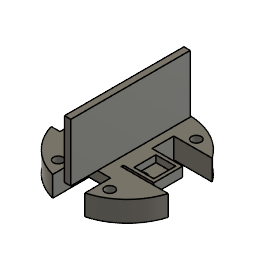
TwoSiPM_Metalens_Holder (Autodesk Fusion 360 design; units mm, degrees)
part number: 2026-07-10-10-46-46-883
Autodesk Fusion 360 part; units mm, degrees
note: some values were not read from the file. Set by a fixed rule: which sketch regions a step uses.
sketch "Sketch Base" plane through (0, 0, 0) normal (0, 1, 0) x (1, 0, 0)
  circle A0 centre (0, 0) radius 19
  line L0 (-4.9826, -7.0157) -> (5.0174, -6.9909)
  line L1 (-4.9826, -7.0157) -> (-4.9545, -18.3427)
  line L2 (5.0174, -6.9909) -> (5.0455, -18.3178)
  line L3 (3.5525, 10.9149) -> (15.552, 10.9149)
  line L4 (-3.5525, 10.9149) -> (-15.552, 10.9149)
  line L5 (3.5525, -5.4945) -> (18.1991, -5.4582)
  line L6 (-3.5525, -5.5769) -> (-18.1631, -5.5769)
  line L7 (3.5525, -5.4945) -> (3.5525, 10.9149)
  line L8 (-3.5525, -5.5769) -> (-3.5525, 10.9149)
  dimension "d1" = 38
  dimension "d4" = 10
  dimension "d10" = 1.5
  dimension "d11" = 7.105
  dimension "d31" = 11.327
  constraint coincident A0.centre origin
  constraint coincident A0 L1.end
  constraint perpendicular L0 L1
  constraint coincident A0 L2.end
  constraint perpendicular L0 L2
  constraint coincident A0 L3.end
  constraint coincident A0 L4.end
  constraint coincident A0 L5.end
  constraint coincident A0 L6.end
  constraint perpendicular L3 L7
  constraint perpendicular L4 L8
  constraint equal L1 L2
  measures "d1" diameter of A0
  measures "d4" distance of L0.start L0.end
  measures "d10" distance of L0 L5
  measures "d11" distance of L7 L8
  measures "d31" distance of L0.start L1.end
extrude "Extrude Base" add sketch "Sketch Base" along normal blind 6.45 contours A0 L0 L1 L2 L3 L4 L5 L6 L7 L8
sketch "Sketch Middle Separations" plane through (0, 6.45, 0) normal (0, 1, 0) x (-1, 0, 0)
  arc A0 (18.1631, 5.5769) -> (4.9545, 18.3427) centre (0, 0) ccw
  line L0 (4.9545, 18.3427) -> (4.9826, 7.0157)
  line L1 (4.9826, 7.0157) -> (-5.0174, 6.9909)
  line L2 (-5.0174, 6.9909) -> (-5.0455, 18.3178)
  arc A1 (-5.0455, 18.3178) -> (-18.1991, 5.4582) centre (0, 0) ccw
  line L3 (-18.1991, 5.4582) -> (-3.5525, 5.4945)
  line L4 (-3.5525, 5.4945) -> (-3.5525, -10.9149)
  line L5 (-3.5525, -10.9149) -> (-15.552, -10.9149)
  arc A2 (-15.552, -10.9149) -> (15.552, -10.9149) centre (0, 0) ccw
  line L6 (15.552, -10.9149) -> (3.5525, -10.9149)
  line L7 (3.5525, -10.9149) -> (3.5525, 5.5769)
  line L8 (3.5525, 5.5769) -> (18.1631, 5.5769)
  line L9 (1, 18.6355) -> (-1, 18.6355)
  line L10 (-1, 18.6355) -> (-1, -18.6355)
  line L11 (1, 18.6355) -> (1, -18.6355)
  line L12 (-1, -18.6355) -> (1, -18.6355)
  line L13 (1, -18.6355) -> (2.1, -18.6355)
  line L14 (2.1, -18.6355) -> (2.1, 10.3085)
  line L15 (2.1, 10.3085) -> (1, 10.3085)
  line L16 (-2.1, -18.6355) -> (-1, -18.6355)
  line L17 (-2.1, -18.6355) -> (-2.1, 10.3085)
  line L18 (-2.1, 10.3085) -> (-1, 10.3085)
  dimension "d15" = 2
  dimension "d16" = 37.271
  dimension "d32" = 28.944
  dimension "d100" = 1.1
  dimension "d114" = 1.1
  constraint perpendicular L9 L10
  constraint perpendicular L9 L11
  constraint equal L10 L11
  constraint perpendicular L11 L13
  constraint perpendicular L13 L14
  constraint coincident L11 L15.end
  constraint perpendicular L11 L15
  constraint perpendicular L10 L16
  constraint perpendicular L5 L17
  constraint coincident L10 L18.end
  constraint perpendicular L10 L18
  constraint equal L14 L17
  measures "d15" distance of L9.start L9.end
  measures "d16" distance of L9.end L10.end
  measures "d32" distance of L16.start L17.end
  measures "d100" distance of L17.end L18.end
  measures "d114" distance of L14.end L15.end
extrude "Extrude Middle Separations" add sketch "Sketch Middle Separations" along normal blind 18 contours L1 L10 L11 L12 | L1 L9 L10 L11
sketch "Sketch Aesthetic" plane through (0.0174, 0, 7.0033) normal (0.002481, 0, 0.999997) x (0.999997, 0, -0.002481)
  line L0 (-5, 0) -> (5, 0)
  line L1 (5, 0) -> (5, 6.45)
  line L2 (5, 6.45) -> (0.9826, 6.45)
  line L3 (0.9826, 6.45) -> (-1.0174, 6.45)
  line L4 (-1.0174, 6.45) -> (-5, 6.45)
  line L5 (-5, 6.45) -> (-5, 0)
  line L6 (5, 6.45) -> (5, 3.35)
  line L7 (5, 3.35) -> (-5, 3.35)
  line L8 (-5, 3.35) -> (-5, 6.45)
  line L9 (5, 6.45) -> (-5, 6.45)
  dimension "d28" = 3.1
  constraint coincident L1.end L2.start
  constraint perpendicular L2 L6
  constraint coincident L5 L7.end
  constraint perpendicular L5 L7
  constraint coincident L4.end L5.start
  measures "d28" distance of L1.end L6.end
extrude "Extrude Aesthetic" add sketch "Sketch Aesthetic" along normal blind 3.3 contours L1 L2 L3 L4 L5 L6 L7 L8 L9
sketch "Sketch 6x6 SiPM Holder" plane through (-3.5525, 0, 0) normal (-1, 0, 0) x (0, 0, 1)
  line L0 (5.5769, 3.45) -> (-5.5301, 3.45)
  line L1 (-5.5301, 3.45) -> (-5.5301, 6.45)
  line L2 (-5.5301, 6.45) -> (5.5769, 6.45)
  line L3 (5.5769, 6.45) -> (5.5769, 3.45)
  line L4 (-10.9149, 0) -> (5.5769, 0)
  line L5 (5.5769, 0) -> (5.5769, 6.45)
  line L6 (5.5769, 6.45) -> (-10.9149, 6.45)
  line L7 (-10.9149, 6.45) -> (-10.9149, 0)
  dimension "d135" = 3
  dimension "d136" = 11.107
  constraint horizontal L0
  constraint vertical L1
  constraint horizontal L2
  constraint vertical L3
  constraint coincident L2.end L6
  constraint coincident L2.end L3.start
  measures "d135" distance of L0.start L2.end
  measures "d136" distance of L0.start L0.end
extrude "Extrude 6x6 SiPM Holder" add sketch "Sketch 6x6 SiPM Holder" along normal blind 11.884 contours L0 L1 L2 L3 L5 L6
sketch "Sketch 6x6 SiPM Holder Bis" plane through (0, 6.45, 0) normal (0, 1, 0) x (-1, 0, 0)
  line L0 (3.5525, -5.5301) -> (15.4365, -5.5301)
  line L1 (15.4365, -5.5301) -> (15.4365, 5.5769)
  line L2 (14.3365, -4.4301) -> (3.5525, -4.4301)
  line L3 (3.5525, -4.4301) -> (3.5525, 4.6399)
  line L4 (3.5525, 4.6399) -> (14.3365, 4.6399)
  line L5 (14.3365, 4.6399) -> (14.3365, -4.4301)
  line L6 (1, -18.6355) -> (-1, -18.6355)
  line L7 (-1, 10.3009) -> (-5.0256, 10.2909)
  line L8 (-5.0256, 10.2909) -> (-5.0455, 18.3178)
  arc A0 (-5.0455, 18.3178) -> (-18.1991, 5.4582) centre (0, 0) ccw
  line L9 (-18.1991, 5.4582) -> (-3.5525, 5.4945)
  line L10 (-3.5525, 5.4945) -> (-3.5525, -10.9149)
  line L11 (-3.5525, -10.9149) -> (-15.552, -10.9149)
  arc A1 (-15.552, -10.9149) -> (15.552, -10.9149) centre (0, 0) ccw
  line L12 (15.552, -10.9149) -> (3.5525, -10.9149)
  line L13 (3.5525, -10.9149) -> (3.5525, -5.5301)
  line L14 (15.4365, 5.5769) -> (18.1631, 5.5769)
  arc A2 (18.1631, 5.5769) -> (4.9545, 18.3427) centre (0, 0) ccw
  line L15 (4.9545, 18.3427) -> (4.9744, 10.3157)
  line L16 (-1, -18.6355) -> (-1, 10.3009)
  line L17 (4.9744, 10.3157) -> (1, 10.3058)
  line L18 (1, 10.3058) -> (1, -18.6355)
  dimension "d142" = 9.07
  dimension "d143" = 10.784
  dimension "d144" = 1.1
  constraint horizontal L2
  constraint vertical L3
  constraint horizontal L4
  constraint vertical L5
  measures "d142" distance of L2.start L4.end
  measures "d143" distance of L3.end L4.end
  measures "d144" distance of L0 L2
extrude "Extrude 6x6 SiPM Holder Bis" cut sketch "Sketch 6x6 SiPM Holder Bis" against normal blind 2.1 contours L2 L3 L4 L5
sketch "Sketch 6x6 SiPM Legs Holes" plane through (0, 4.35, 0) normal (0, 1, 0) x (-1, 0, 0)
  line L0 (3.5525, -4.4304) -> (14.3365, -4.4304)
  line L1 (14.3365, -4.4304) -> (14.3365, 4.6396)
  line L2 (14.3365, 4.6396) -> (3.5525, 4.6396)
  line L3 (3.5525, 4.6396) -> (3.5525, -4.4304)
  circle A0 centre (5.3481, 0.1396) radius 1
  circle A1 centre (12.7861, 0.1396) radius 1
  line L4 (14.3365, 4.6399) -> (3.5525, 4.6399)
  line L5 (3.5525, 4.6399) -> (3.5525, -4.4301)
  line L6 (3.5525, -4.4301) -> (14.3365, -4.4301)
  line L7 (14.3365, -4.4301) -> (14.3365, 4.6399)
  circle A2 centre (5.3481, 2.3396) radius 1
  line L8 (4.3481, 2.3396) -> (4.3481, 0.1396)
  line L9 (6.3481, 2.3349) -> (6.3481, 0.1396)
  circle A3 centre (12.7861, 2.3396) radius 1
  line L10 (11.7861, 2.3396) -> (11.7861, 0.1396)
  line L11 (13.7861, 2.3396) -> (13.7855, 0.1046)
  dimension "d63" = 2
  dimension "d67" = 4.5
  dimension "d95" = 2
  dimension "d96" = 7.438
  dimension "d152" = 2
  dimension "d153" = 2.2
  dimension "d154" = 2.3
  dimension "d155" = 2
  constraint coincident A1 L11.end
  constraint coincident A2 L8.start
  constraint coincident A0 L8.end
  constraint tangent A0 L8
  constraint coincident A2 L9.start
  constraint coincident A0 L9.end
  constraint tangent A0 L9
  constraint coincident A3 L10.start
  constraint coincident A1 L10.end
  constraint tangent A1 L10
  constraint vertical L10
  constraint coincident A3 L11.start
  measures "d63" diameter of A0
  measures "d67" distance of L2 A0.centre
  measures "d95" diameter of A1
  measures "d96" distance of A0.centre A1.centre
  measures "d152" diameter of A2
  measures "d153" distance of A0.centre A2.centre
  measures "d154" distance of L2 A2.centre
  measures "d155" diameter of A3
extrude "Extrude 6x6 SiPM Legs Holes" cut sketch "Sketch 6x6 SiPM Legs Holes" against normal blind 1.1 contours A0 | A0 A2 L8 L9 | A2 | A1 L11 | A1 A3 L10 L11 | A3
sketch "Sketch 3x3 SiPM Holder" plane through (3.5525, 0, 0) normal (1, 0, 0) x (0, 0, -1)
  line L0 (-5.4945, 0) -> (10.9149, 0)
  line L1 (10.9149, 0) -> (10.9149, 6.45)
  line L2 (10.9149, 6.45) -> (-5.4945, 6.45)
  line L3 (-5.4945, 6.45) -> (-5.4945, 0)
  line L4 (-4.83, 6.45) -> (4.17, 6.45)
  line L5 (4.17, 6.45) -> (4.17, 3.45)
  line L6 (4.17, 3.45) -> (-4.83, 3.45)
  line L7 (-4.83, 3.45) -> (-4.83, 6.45)
  dimension "d148" = 3
  dimension "d149" = 9
  constraint horizontal L4
  constraint vertical L5
  constraint horizontal L6
  constraint vertical L7
  measures "d148" distance of L4.start L6.end
  measures "d149" distance of L5.end L6.end
extrude "Extrude 3x3 SiPM Holder (1)" add sketch "Sketch 3x3 SiPM Holder" along normal blind 9.517 contours L2 L4 L5 L6 L7
sketch "Sketch 3x3 SiPM Holder Bis" plane through (0, 6.45, 0) normal (0, 1, 0) x (-1, 0, 0)
  line L0 (2.1, 10.3085) -> (2.1, -18.6355)
  line L1 (2.1, -18.6355) -> (-2.1, -18.6355)
  line L2 (-2.1, -18.6355) -> (-2.1, 10.2981)
  line L3 (-2.1, 10.2981) -> (-5.0256, 10.2909)
  line L4 (-5.0256, 10.2909) -> (-5.0455, 18.3178)
  arc A0 (-5.0455, 18.3178) -> (-18.1991, 5.4582) centre (0, 0) ccw
  line L5 (-18.1991, 5.4582) -> (-3.5525, 5.4945)
  line L6 (-3.5525, 5.4945) -> (-3.5525, -10.9149)
  line L7 (-3.5525, -10.9149) -> (-15.552, -10.9149)
  arc A1 (-15.552, -10.9149) -> (15.552, -10.9149) centre (0, 0) ccw
  line L8 (15.552, -10.9149) -> (3.5525, -10.9149)
  line L9 (3.5525, -10.9149) -> (3.5525, 5.5769)
  line L10 (3.5525, 5.5769) -> (18.1631, 5.5769)
  arc A2 (18.1631, 5.5769) -> (4.9545, 18.3427) centre (0, 0) ccw
  line L11 (4.9545, 18.3427) -> (4.9744, 10.3157)
  line L12 (4.9744, 10.3157) -> (2.0818, 10.3085)
  line L13 (2.0818, 10.3085) -> (2.1, 10.3085)
  line L14 (-11.9695, 3.73) -> (-5.8195, 3.73)
  line L15 (-11.9695, 3.73) -> (-11.9695, -3.07)
  line L16 (-11.9695, -3.07) -> (-5.8195, -3.07)
  line L17 (-5.8195, -3.07) -> (-5.8195, 3.73)
  line L18 (-3.5525, 4.83) -> (-13.0695, 4.83)
  line L19 (-13.0695, 4.83) -> (-13.0695, -4.17)
  line L20 (-13.0695, -4.17) -> (-3.5525, -4.17)
  line L21 (-3.5525, 5.4945) -> (-3.5525, 4.83)
  line L22 (1, -18.6355) -> (-1, -18.6355)
  line L23 (-1, 10.3009) -> (-5.0256, 10.2909)
  line L24 (-5.0256, 10.2909) -> (-5.0455, 18.3178)
  arc A3 (-5.0455, 18.3178) -> (-18.1991, 5.4582) centre (0, 0) ccw
  line L25 (-18.1991, 5.4582) -> (-3.5525, 5.4945)
  line L26 (-3.5525, -4.17) -> (-3.5525, -10.9149)
  line L27 (-3.5525, -10.9149) -> (-15.552, -10.9149)
  arc A4 (-15.552, -10.9149) -> (15.552, -10.9149) centre (0, 0) ccw
  line L28 (15.552, -10.9149) -> (3.5525, -10.9149)
  line L29 (3.5525, -10.9149) -> (3.5525, -5.5301)
  line L30 (3.5525, -4.4301) -> (3.5525, 4.6399)
  line L31 (15.4365, 5.5769) -> (18.1631, 5.5769)
  arc A5 (18.1631, 5.5769) -> (4.9545, 18.3427) centre (0, 0) ccw
  line L32 (4.9545, 18.3427) -> (4.9744, 10.3157)
  line L33 (3.5525, 4.6399) -> (14.3365, 4.6399)
  line L34 (14.3365, 4.6399) -> (14.3365, -4.4301)
  line L35 (14.3365, -4.4301) -> (3.5525, -4.4301)
  line L36 (3.5525, -5.5301) -> (15.4365, -5.5301)
  line L37 (15.4365, -5.5301) -> (15.4365, 5.5769)
  line L38 (-1, -18.6355) -> (-1, 10.3009)
  line L39 (4.9744, 10.3157) -> (1, 10.3058)
  line L40 (1, 10.3058) -> (1, -18.6355)
  dimension "d78" = 6.15
  dimension "d82" = 6.8
  constraint perpendicular L15 L16
  constraint equal L14 L16
  measures "d78" distance of L14.start L14.end
  measures "d82" distance of L14.start L15.end
extrude "Extrude 3x3 SiPM Holder Bis" cut sketch "Sketch 3x3 SiPM Holder Bis" against normal blind 2.1 contours L14 L15 L16 L17
sketch "Sketch 3x3 SiPM Legs Holes" plane through (0, 4.35, 0) normal (0, 1, 0) x (-1, 0, 0)
  line L0 (-11.9695, 3.73) -> (-11.9695, -3.07)
  line L1 (-11.9695, -3.07) -> (-5.8195, -3.07)
  line L2 (-5.8195, -3.07) -> (-5.8195, 3.73)
  line L3 (-5.8195, 3.73) -> (-11.9695, 3.73)
  circle A0 centre (-10.1695, 2.33) radius 1
  circle A1 centre (-7.6195, 2.33) radius 1
  line L4 (-11.9695, 3.73) -> (-11.9695, -3.07)
  line L5 (-11.9695, -3.07) -> (-5.8195, -3.07)
  line L6 (-5.8195, -3.07) -> (-5.8195, 3.73)
  line L7 (-5.8195, 3.73) -> (-11.9695, 3.73)
  circle A2 centre (-6.8295, 2.33) radius 1
  line L8 (-7.6213, 3.33) -> (-6.8295, 3.33)
  line L9 (-7.6213, 1.33) -> (-6.8295, 1.33)
  circle A3 centre (-10.9595, 2.33) radius 1
  line L10 (-10.1684, 3.33) -> (-10.9595, 3.33)
  line L11 (-10.9595, 1.33) -> (-10.1695, 1.33)
  dimension "d85" = 2
  dimension "d87" = 2.55
  dimension "d158" = 2
  dimension "d160" = 2
  dimension "d161" = 0.79
  dimension "d162" = 0.79
  constraint coincident A1 L8.start
  constraint coincident A2 L8.end
  constraint tangent A2 L8
  constraint coincident A1 L9.start
  constraint coincident A2 L9.end
  constraint tangent A2 L9
  constraint coincident A0 L10.start
  constraint coincident A3 L10.end
  constraint tangent A3 L10
  constraint coincident A3 L11.start
  constraint coincident A0 L11.end
  constraint tangent A0 L11
  constraint horizontal L11
  measures "d85" diameter of A0
  measures "d87" horizontal distance of A0.centre A1.centre
  measures "d158" diameter of A2
  measures "d160" diameter of A3
  measures "d161" distance of A0.centre A3.centre
  measures "d162" distance of A1.centre A2.centre
extrude "Extrude 3x3 SiPM Legs Holes" cut sketch "Sketch 3x3 SiPM Legs Holes" against normal blind 1.1 contours A0 A3 L10 | A0 A3 | A0 A3 L11 | A0 A3 | A0 A3 | A1 A2 L9 | A1 A2 | A1 A2 L8 | A1 A2 | A1 A2
sketch "Sketch Base Crews Holes" plane through (0, 6.45, 0) normal (0, 1, 0) x (-1, 0, 0)
  line L0 (1, -18.6355) -> (-1, -18.6355)
  line L1 (-1, 10.3009) -> (-5.0256, 10.2909)
  line L2 (-5.0256, 10.2909) -> (-5.0455, 18.3178)
  arc A0 (-5.0455, 18.3178) -> (-18.1991, 5.4582) centre (0, 0) ccw
  line L3 (-18.1991, 5.4582) -> (-3.5525, 5.4945)
  line L4 (-3.5525, 5.4945) -> (-3.5525, 4.83)
  line L5 (-3.5525, -10.9149) -> (-15.552, -10.9149)
  arc A1 (-15.552, -10.9149) -> (15.552, -10.9149) centre (0, 0) ccw
  line L6 (15.552, -10.9149) -> (3.5525, -10.9149)
  line L7 (3.5525, -10.9149) -> (3.5525, -5.5301)
  line L8 (15.4365, 5.5769) -> (18.1631, 5.5769)
  arc A2 (18.1631, 5.5769) -> (4.9545, 18.3427) centre (0, 0) ccw
  line L9 (4.9545, 18.3427) -> (4.9744, 10.3157)
  circle A3 centre (8.0047, 13.5403) radius 1.5
  circle A4 centre (-7.9953, 13.5006) radius 1.5
  circle A5 centre (-7.9281, -13.5711) radius 1.5
  circle A6 centre (8.0719, -13.5711) radius 1.5
  line L10 (-5.8195, -3.07) -> (-11.9695, -3.07)
  line L11 (-11.9695, -3.07) -> (-11.9695, 3.73)
  line L12 (-11.9695, 3.73) -> (-5.8195, 3.73)
  line L13 (-5.8195, 3.73) -> (-5.8195, -3.07)
  line L14 (-3.5525, 4.83) -> (-13.0695, 4.83)
  line L15 (-13.0695, 4.83) -> (-13.0695, -4.17)
  line L16 (-13.0695, -4.17) -> (-3.5525, -4.17)
  line L17 (-3.5525, -4.17) -> (-3.5525, -10.9149)
  line L18 (3.5525, -4.4301) -> (3.5525, 4.6399)
  line L19 (3.5525, 4.6399) -> (14.3365, 4.6399)
  line L20 (14.3365, 4.6399) -> (14.3365, -4.4301)
  line L21 (14.3365, -4.4301) -> (3.5525, -4.4301)
  line L22 (3.5525, -5.5301) -> (15.4365, -5.5301)
  line L23 (15.4365, -5.5301) -> (15.4365, 5.5769)
  line L24 (-1, -18.6355) -> (-1, 10.3009)
  line L25 (4.9744, 10.3157) -> (1, 10.3058)
  line L26 (1, 10.3058) -> (1, -18.6355)
  dimension "d104" = 3
  dimension "d105" = 16
  dimension "d107" = 3
  dimension "d111" = 3
  dimension "d113" = 3
  dimension "d126" = 27.0717
  measures "d104" diameter of A3
  measures "d105" distance of A3.centre A4.centre
  measures "d107" diameter of A4
  measures "d111" diameter of A5
  measures "d113" diameter of A6
  measures "d126" vertical distance of A4.centre A5.centre
extrude "Extrude Base Crews Holes" cut sketch "Sketch Base Crews Holes" against normal blind 7.7 contours A3 | A4 | A5 | A6
